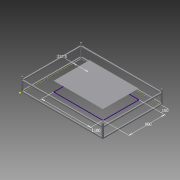
# Autodesk Inventor part: CloudGraffitiPlotterRig
Saved by Autodesk Inventor 2014 SP1 (Build 180222100, 222)
## iProperties
Created: 2017-02-12
Part Number: CloudGraffitiPlotterRig
Material: Generic
Document SubType Name: Modeling
Designer: danielsikar
Density: 1 g/cm^3
Appearance: Default
Author: danielsikar
Autodesk Inventor part; units mm, degrees
ref_plane "YZ Plane" through (0, 0, 0) normal (1, 0, 0) x (0, 1, 0)
sketch "Sketch1" plane through (0, 0, 0) normal (0, 0, 1) x (1, 0, 0)
  line L0 (0, 0) -> (29.7379, 0) construction
  line L1 (0, 1340) -> (25, 1340)
  line L2 (25, 1340) -> (25, 1365)
  line L3 (25, 1365) -> (0, 1365)
  line L4 (0, 1365) -> (0, 1340)
  line L5 (1800, 1365) -> (1825, 1365)
  line L6 (1825, 1365) -> (1825, 1340)
  line L7 (1825, 1340) -> (1800, 1340)
  line L8 (1800, 1340) -> (1800, 1365)
  line L9 (1734.4226, 849.9895) -> (1993.1274, 849.9895) construction
  dimension "d0" = 25
  dimension "d1" = 25
  dimension "d2" = 1340
  dimension "d3" = 25
  dimension "d4" = 25
  dimension "d5" = 1800
  dimension "d6" = 490.0105
  dimension "d7" = 1340
  constraints: 20 end point, 4 parallel, 3 horizontal, 3 perpendicular
  measures "d0" distance of L3.end L2.end
  measures "d1" distance of L2.end L1.end
  measures "d2" distance between parallel lines of L0 L1
  measures "d3" distance of L6.end L7.end
  measures "d4" distance of L5.end L6.end
  measures "d5" distance from line of L8 L0.start
  measures "d6" distance between parallel lines of L9 L7
  measures "d7" distance from line of L7 L0.start
extrude "Extrusion1" add sketch "Sketch1" along normal blind 300
sketch "Sketch2" plane through (0, 1340, 0) normal (0, -1, 0) x (1, 0, 0)
  line L0 (25, 0) -> (25, 300) projected
  line L1 (0, 300) -> (25, 300) projected
  line L2 (0, 0) -> (0, 300) projected
  line L3 (0, 240) -> (25, 240)
  line L4 (25, 240) -> (25, 215)
  line L5 (25, 215) -> (0, 215)
  line L6 (0, 215) -> (0, 240)
  dimension "d10" = 25
  dimension "d11" = 60
  constraints: 8 end point, 2 parallel, 2 point on line, 1 horizontal, 1 perpendicular
  measures "d10" distance between parallel lines of L5 L3
  measures "d11" distance between parallel lines of L3 L1
extrude "Extrusion2" add sketch "Sketch2" along normal blind 1315 contours L5 L2 L3 L0
sketch "Sketch4" plane through (0, 25, 240) normal (0, 0, 1) x (1, 0, 0)
  line L0 (25, 1315) -> (25, 0) projected
  line L1 (0, 0) -> (25, 0)
  line L2 (25, 0) -> (25, 25)
  line L3 (25, 25) -> (0, 25)
  line L4 (0, 25) -> (0, 0)
  point P0 (0, -25)
  dimension "d14" = 25
  constraints: 8 end point, 2 parallel, 1 horizontal, 1 perpendicular, 1 point on line
  measures "d14" distance of L2.end L1.end
extrude "Extrusion3" add sketch "Sketch4" along normal up to surface (60 mm away)
sketch "Sketch5" plane through (25, 25, 215) normal (0, 0, -1) x (-1, 0, 0)
  line L0 (25, 1315) -> (25, 0) projected
  line L1 (0, 0) -> (25, 0)
  line L2 (25, 0) -> (25, 25)
  line L3 (25, 25) -> (0, 25)
  line L4 (0, 25) -> (0, 0)
  point P0 (25, -25)
  dimension "d17" = 25
  constraints: 8 end point, 2 parallel, 1 horizontal, 1 perpendicular, 1 point on line
  measures "d17" distance of L2.end L1.end
extrude "Extrusion4" add sketch "Sketch5" along normal up to surface (215 mm away)
sketch "Sketch6" plane through (0, 50, 215) normal (0, 1, 0) x (1, 0, 0)
  line L0 (25, 0) -> (25, 215) projected
  line L1 (0, 215) -> (25, 215)
  line L2 (25, 215) -> (25, 190)
  line L3 (25, 190) -> (0, 190)
  line L4 (0, 190) -> (0, 215)
  dimension "d20" = 25
  constraints: 8 end point, 2 parallel, 1 horizontal, 1 perpendicular, 1 point on line
  measures "d20" distance of L1.end L2.end
extrude "Extrusion5" add sketch "Sketch6" along normal up to surface (1290 mm away)
sketch "Sketch7" plane through (25, 1365, 300) normal (1, 0, 0) x (0, 0, -1)
  line L0 (275, -25) -> (300, -25)
  line L1 (300, -25) -> (300, 0)
  line L2 (300, 0) -> (275, 0)
  line L3 (275, 0) -> (275, -25)
  point P0 (300, -1365)
  constraints: 8 end point, 2 parallel, 1 horizontal, 1 perpendicular
extrude "Extrusion6" add sketch "Sketch7" along normal up to surface (1775 mm away)
sketch "Sketch8" plane through (25, 25, 0) normal (1, 0, 0) x (0, 0, -1)
  line L0 (-25, 1340) -> (-300, 1340) projected
  line L1 (-215, 1315) -> (-240, 1315)
  line L2 (-240, 1315) -> (-240, 1340)
  line L3 (-240, 1340) -> (-215, 1340)
  line L4 (-215, 1340) -> (-215, 1315)
  point P0 (0, -25)
  constraints: 8 end point, 2 parallel, 1 horizontal, 1 perpendicular, 1 point on line
extrude "Extrusion7" add sketch "Sketch8" along normal up to surface (1775 mm away)
ref_plane "Work Plane1" through (912.5, 1365, 0) normal (-1, 0, 0) x (0, 0, 1)
mirror "Mirror1" about plane through (912.5, 1365, 0) normal (-1, 0, 0) of "Extrusion2", "Extrusion3", "Extrusion4", "Extrusion5"
ref_plane "Work Plane2" through (1800, 695, 0) normal (0, -1, 0) x (1, 0, 0)
mirror "Mirror2" about plane through (1800, 695, 0) normal (0, -1, 0) of "Extrusion7", "Extrusion6"
sketch "Sketch9" plane through (0, 0, 0) normal (0, 0, 1) x (1, 0, 0)
  line L0 (25, 1340) -> (1800, 1340) construction
  line L1 (1800, 1340) -> (1800, 50) construction
  line L2 (25, 1340) -> (25, 50) construction
  line L3 (362.5, 1190) -> (1462.5, 1190)
  line L4 (1462.5, 1190) -> (1462.5, 390)
  line L5 (1462.5, 390) -> (362.5, 390)
  line L6 (362.5, 390) -> (362.5, 1190)
  line L7 (25, 50) -> (1800, 50) construction
  point P0 (0, 0)
  dimension "d29" = 800
  dimension "d30" = 1100
  dimension "d31" = 337.5
  dimension "d33" = 150
  constraints: 8 end point, 2 parallel, 1 horizontal, 1 perpendicular
  measures "d29" distance between parallel lines of L5 L3
  measures "d30" distance between parallel lines of L4 L6
  measures "d31" distance between parallel lines of L6 L2
  measures "d33" distance between parallel lines of L3 L0
sketch "Sketch10" plane through (1825, 50, 215) normal (0, 0, -1) x (-1, 0, 0)
  line L0 (362.5, 340) -> (1462.5, 340) projected
  line L1 (1462.5, 340) -> (1462.5, 1140) projected
  line L2 (1462.5, 1140) -> (362.5, 1140) projected
  line L3 (362.5, 1140) -> (362.5, 340) projected
  point P0 (1825, -50)
extrude "Extrusion8" add sketch "Sketch10" along normal blind 2
body "Solid1"
